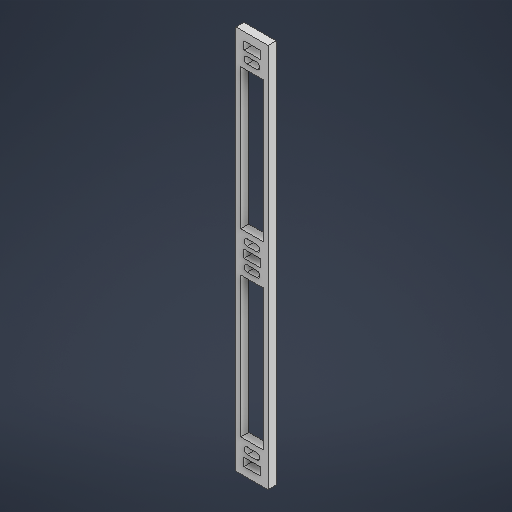
# Autodesk Inventor part: base botellas
Saved by Autodesk Inventor 2025.3 (Build 293356000, 356)
## iProperties
Created: 2025-11-02
Part Number: base botellas
Material: Generic
Document SubType Name: Modeling
Designer: santi
Density: 1 g/cm^3
Appearance: Default
Author: santi
Autodesk Inventor part; units mm, degrees
ref_plane "YZ Plane" through (0, 0, 0) normal (1, 0, 0) x (0, 1, 0)
ref_plane "XZ Plane" through (0, 0, 0) normal (0, 1, 0) x (-1, 0, 0)
ref_plane "XY Plane" through (0, 0, 0) normal (0, 0, 1) x (1, 0, 0)
sketch "Sketch1" plane through (0, 0, 0) normal (0, 0, 1) x (1, 0, 0)
  line L0 (-10, 120) -> (10, 120)
  line L1 (10, 120) -> (10, -120)
  line L2 (10, -120) -> (-10, -120)
  line L3 (-10, -120) -> (-10, 120)
  line L4 (0, 0) -> (10, 0) construction
  line L5 (-5, 2.5) -> (5, 2.5)
  line L6 (5, 2.5) -> (5, -2.5)
  line L7 (5, -2.5) -> (-5, -2.5)
  line L8 (-5, -2.5) -> (-5, 2.5)
  line L9 (-5, -110) -> (5, -110)
  line L10 (5, -110) -> (5, -115)
  line L11 (5, -115) -> (-5, -115)
  line L12 (-5, -115) -> (-5, -110)
  line L13 (-5, 110) -> (5, 110)
  line L14 (5, 110) -> (5, 115)
  line L15 (5, 115) -> (-5, 115)
  line L16 (-5, 115) -> (-5, 110)
  line L17 (-3, 7) -> (3, 7) construction
  line L18 (-3, 5) -> (3, 5)
  line L19 (3, 9) -> (-3, 9)
  arc A0 (-3, 9) -> (-3, 5) centre (-3, 7) ccw
  arc A1 (3, 5) -> (3, 9) centre (3, 7) ccw
  line L20 (-3, 105.5) -> (3, 105.5) construction
  line L21 (-3, 103.5) -> (3, 103.5)
  line L22 (3, 107.5) -> (-3, 107.5)
  arc A2 (-3, 107.5) -> (-3, 103.5) centre (-3, 105.5) ccw
  arc A3 (3, 103.5) -> (3, 107.5) centre (3, 105.5) ccw
  line L23 (-3, -7) -> (3, -7) construction
  line L24 (-3, -9) -> (3, -9)
  line L25 (3, -5) -> (-3, -5)
  arc A4 (-3, -5) -> (-3, -9) centre (-3, -7) ccw
  arc A5 (3, -9) -> (3, -5) centre (3, -7) ccw
  line L26 (-3, -105.5) -> (3, -105.5) construction
  line L27 (-3, -107.5) -> (3, -107.5)
  line L28 (3, -103.5) -> (-3, -103.5)
  arc A6 (-3, -103.5) -> (-3, -107.5) centre (-3, -105.5) ccw
  arc A7 (3, -107.5) -> (3, -103.5) centre (3, -105.5) ccw
  line L29 (-7, 100) -> (7, 100)
  line L30 (7, 100) -> (7, 12.5)
  line L31 (7, 12.5) -> (-7, 12.5)
  line L32 (-7, 12.5) -> (-7, 100)
  line L33 (-7, -12.5) -> (7, -12.5)
  line L34 (7, -12.5) -> (7, -100)
  line L35 (7, -100) -> (-7, -100)
  line L36 (-7, -100) -> (-7, -12.5)
  point P0 (0, 120)
  point P1 (10, 0)
  point P2 (5, 0)
  point P3 (0, -2.5)
  point P4 (5, 0)
  point P5 (0, 7)
  point P6 (0, 105.5)
  point P7 (0, -7)
  point P8 (0, -105.5)
  dimension "d0" = 240
  dimension "d1" = 20
  dimension "d2" = 10
  dimension "d3" = 5
  dimension "d4" = 107.5
  dimension "d5" = 5
  dimension "d6" = 5
  dimension "d7" = 5
  dimension "d10" = 2
  dimension "d11" = 2.5
  dimension "d12" = 7
  dimension "d13" = 7
  dimension "d14" = 2.5
  dimension "d15" = 2
  dimension "d16" = 7
  dimension "d17" = 7
  dimension "d18" = 2
  dimension "d19" = 6
  dimension "d20" = 7
  dimension "d21" = 2.5
  dimension "d22" = 2.5
  dimension "d23" = 2
  dimension "d24" = 7
  dimension "d25" = 7
  dimension "d28" = 3.5
  dimension "d29" = 3.5
  dimension "d30" = 3
  dimension "d31" = 3
  dimension "d32" = 3.5
  dimension "d33" = 3.5
  dimension "d34" = 3
  dimension "d35" = 3
  constraints: 82 end point, 16 point on circle, 16 tangent, 14 parallel, 10 midpoint, 9 horizontal, 8 centre point, 6 perpendicular, 4 symmetric about line, 2 horizontal alignment, 2 vertical alignment
  measures "d0" distance of L0.end L1.end
  measures "d1" distance of L1.end L2.end
  measures "d2" distance of L6.end L7.end
  measures "d3" distance of L5.end L6.end
  measures "d4" distance between parallel lines of L9 L7
  measures "d5" distance of L9.end L10.end
  measures "d6" distance between parallel lines of L3 L12
  measures "d7" distance between parallel lines of L1 L10
  measures "d10" radius of A1
  measures "d11" distance between parallel lines of L5 L18
  measures "d12" distance from line of L1 L17.end
  measures "d13" distance from line of L3 L17.start
  measures "d14" distance between parallel lines of L13 L22
  measures "d15" radius of A3
  measures "d16" distance from line of L1 L20.end
  measures "d17" distance from line of L3 L20.start
  measures "d18" radius of A5
  measures "d19" distance of L24.start L24.end
  measures "d20" distance from line of L3 L23.start
  measures "d21" distance between parallel lines of L7 L25
  measures "d22" distance between parallel lines of L9 L27
  measures "d23" radius of A7
  measures "d24" distance from line of L1 L26.end
  measures "d25" distance from line of L3 L26.start
  measures "d28" distance between parallel lines of L29 L21
  measures "d29" distance between parallel lines of L19 L31
  measures "d30" distance between parallel lines of L1 L30
  measures "d31" distance between parallel lines of L3 L32
  measures "d32" distance between parallel lines of L24 L33
  measures "d33" distance between parallel lines of L35 L28
  measures "d34" distance between parallel lines of L1 L34
  measures "d35" distance between parallel lines of L3 L36
extrude "Extrusion3" add sketch "Sketch1" along normal blind 5
body "Solid3"
